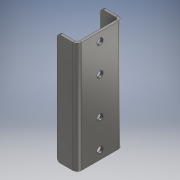
# Autodesk Inventor part: Poot
Saved by Autodesk Inventor 2017 (Build 210142000, 142)
## iProperties
Created: 2017-01-07
Part Number: Poot
Material: Steel, Mild
Document SubType Name: Sheet Metal
Designer: bramp
Density: 7.85 g/cm^3
Sheet Metal Rule: Default_mm
Appearance: Semi-Polished
Author: bramp
Autodesk Inventor part; units mm, degrees
ref_plane "YZ Plane" through (0, 0, 0) normal (1, 0, 0) x (0, 1, 0)
ref_plane "XZ Plane" through (0, 0, 0) normal (0, 1, 0) x (-1, 0, 0)
ref_plane "XY Plane" through (0, 0, 0) normal (0, 0, 1) x (1, 0, 0)
sketch "Sketch1" plane through (0, 0, 0) normal (0, 0, 1) x (1, 0, 0)
  line L0 (-35, 0) -> (0, 0)
  line L1 (0, 0) -> (0, 80)
  line L2 (0, 80) -> (-35, 80)
  dimension "d0" = 35
  dimension "d1" = 35
  dimension "d2" = 80
  measures "d0" distance of L0.start L0.end
  measures "d1" distance of L1.end L2.end
  measures "d2" distance of L0.end L1.end
contour flange "Contour Flange1" sketch "Sketch1" thickness 4 bend radius 3.9 width 195 along (0, 0, 1) mid plane no both sides no wall seen from (-17.5, 0, 0) lies toward (0, 1, 0) curves L0 L1 L2
bend "Bend1"
corner "Corner1"
fillet "Fillet1" radius 5 4 edges at (-35, 2, 195) (-35, 2, 0) (-35, 78, 195) (-35, 78, 0)
sketch "Sketch2" plane through (0, 7.9, 195) normal (1, 0, 0) x (0, 0, -1)
  line L0 (0, 64.2) -> (195, 64.2) projected
  line L1 (0, 0) -> (0, 64.2) projected
  line L2 (0, 0) -> (195, 0) projected
  line L3 (195, 0) -> (195, 64.2) projected
  line L4 (0, 64.2) -> (0, 0) construction
  line L5 (0, 32.1) -> (195, 32.1) construction
  point P0 (195, -7.9)
  point P1 (15, 32.1)
  point P2 (65, 32.1)
  point P3 (130, 32.1)
  point P4 (180, 32.1)
  dimension "d14" = 15
  dimension "d15" = 50
  dimension "d16" = 50
  dimension "d17" = 15
  constraints: 4 point on line, 2 end point, 2 midpoint
  measures "d14" distance from line of L1 point (15, 32.1)
  measures "d15" distance of point (15, 32.1) point (65, 32.1)
  measures "d16" distance of point (180, 32.1) point (130, 32.1)
  measures "d17" distance from line of L3 point (180, 32.1)
hole "Hole1" at (0, 40, 180) at (0, 40, 130) at (0, 40, 65) at (0, 40, 15) direction (-1, 0, 0) diameter 11 end through all
equation "\"d1\" = d0"
equation "\"d23\" = Thickness"
equation "\"d3\" = BendReliefWidth"
equation "\"d4\" = BendReliefDepth"
equation "\"d5\" = MinimumRemnant"
equation "\"d6\" = BendRadius"
equation "\"d8\" = BendRadius"
equation "\"d10\" = CornerReliefSize"
equation "\"d11\" = GapSize"
equation "\"d12\" = JacobiRadiusSize"
equation "\"BendReliefWidth\" = Thickness"
equation "\"BendReliefDepth\" = 0.5 * Thickness"
equation "\"CornerReliefSize\" = 4 * Thickness"
equation "\"MinimumRemnant\" = 2 * Thickness"
equation "\"TransitionRadius\" = BendRadius"
equation "\"JacobiRadiusSize\" = BendRadius"
equation "\"GapSize\" = Thickness"
equation "\"Thickness\" = 4"
equation "\"BendRadius\" = 3.9"
body "Solid1"
